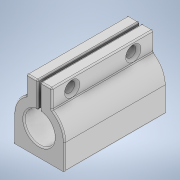
# Autodesk Inventor part: Holder
Saved by Autodesk Inventor 2022 (Build 260153000, 153)
## iProperties
Created: 2022-04-05
Part Number: Holder
Material: Generic
Document SubType Name: Modeling
Designer: thoms
Density: 1 g/cm^3
Appearance: Default
Author: thoms
Autodesk Inventor part; units mm, degrees
ref_plane "YZ Plane" through (0, 0, 0) normal (1, 0, 0) x (0, 1, 0)
ref_plane "XZ Plane" through (0, 0, 0) normal (0, 1, 0) x (-1, 0, 0)
ref_plane "XY Plane" through (0, 0, 0) normal (0, 0, 1) x (1, 0, 0)
sketch "Sketch1" plane through (0, 0, 0) normal (0, 0, 1) x (1, 0, 0)
  arc A0 (-2.5, 4.3301) -> (2.5, 4.3301) centre (0, 0) ccw
  line L0 (2.5, 4.3301) -> (2.5, 8)
  line L1 (2.5, 8) -> (-2.5, 8)
  line L2 (-2.5, 8) -> (-2.5, 4.3301)
  circle A1 centre (0, 0) radius 2.95
  line L3 (-0.25, 8) -> (0.25, 8)
  line L4 (0.25, 8) -> (0.25, 2.5)
  line L5 (0.25, 2.5) -> (-0.25, 2.5)
  line L6 (-0.25, 2.5) -> (-0.25, 8)
  line L7 (-5, 0) -> (-5, -5)
  line L8 (-5, -5) -> (0, -5)
  line L9 (5, 0) -> (5, -5)
  line L10 (5, -5) -> (0, -5)
  point P0 (0.25, 2.9394)
  point P1 (-0.25, 2.9394)
  dimension "d0" = 10
  dimension "d1" = 5
  dimension "d2" = 2.5
  dimension "d3" = 8
  dimension "d4" = 3.6699
  dimension "d7" = 5.9
  dimension "d8" = 0.5
  dimension "d9" = 0.25
  dimension "d10" = 0
  dimension "d11" = 5.5
  constraints: 22 end point, 5 point on circle, 3 parallel, 2 centre point, 2 coincident, 2 perpendicular, 2 vertical, 1 horizontal, 1 tangent
  measures "d0" diameter of A0
  measures "d1" distance of L0.end L1.end
  measures "d2" distance from line of point (0, 0) L0
  measures "d3" distance from line of point (0, 0) L1
  measures "d4" distance of L1.end L2.end
  measures "d7" diameter of A1
  measures "d8" distance of L3.start L3.end
  measures "d9" distance from line of point (0, 0) L4
  measures "d10" distance between parallel lines of L1 L3
  measures "d11" distance of L3.end L4.end
extrude "Extrusion1" add sketch "Sketch1" against normal blind 20 contours L2 L1 L6 A1 L4 L0 A0 | A0 L8 L7 | A0 L9 L10
sketch "Sketch2" plane through (2.5, 4.3301, 0) normal (1, 0, 0) x (0, 0, -1)
  circle A0 centre (4, 1.6699) radius 1
  circle A1 centre (16, 1.6699) radius 1
  line L0 (0, 0) -> (0, 3.6699) projected
  line L1 (20, 3.6699) -> (20, 0) projected
  line L2 (0, 3.6699) -> (20, 3.6699) projected
  point P0 (0, -4.3301)
  dimension "d12" = 2
  dimension "d13" = 4
  dimension "d14" = 2
  dimension "d15" = 4
  dimension "d16" = 2
  dimension "d17" = 2
  constraints: 2 centre point
  measures "d12" diameter of A0
  measures "d13" distance from line of L0 A0.centre
  measures "d14" diameter of A1
  measures "d15" distance from line of L1 A1.centre
  measures "d16" distance from line of L2 A0.centre
  measures "d17" distance from line of L2 A1.centre
extrude "Extrusion2" cut sketch "Sketch2" against normal up to surface (5 mm away)
chamfer "Chamfer1" distance 0.5 angle 45 2 edges at (2.5, 6, -3) (2.5, 6, -15)
fillet "Fillet1" radius 0.25 32 edges at (-0.25, 5.4697, 0) (0.25, 5.4697, 0) (-0.25, 8, -10) (0.25, 8, -10) (-1.375, 8, -20) (1.375, 8, -20) (-0.25, 5.4697, -20) (0.25, 5.4697, -20) (-1.375, 8, 0) (1.375, 8, 0) (-2.5, 8, -10) (-2.5, 6.1651, 0) (-2.5, 6.1651, -20) (2.5, 8, -10) (2.5, 6.1651, -20) (2.5, 6.1651, 0) (-5, -2.5, 0) (-4.3301, 2.5, 0) (5, -2.5, 0) (4.3301, 2.5, 0) (5, -2.5, -20) (4.3301, 2.5, -20) (0, -2.95, 0) (-5, -2.5, -20) (-4.3301, 2.5, -20) (0, -2.95, -20) (0.25, 2.9394, -10) (-0.25, 2.9394, -10) (-2.5, 4.3301, -10) (2.5, 4.3301, -10) (-5, -5, -10) (5, -5, -10)
body "Solid1"
